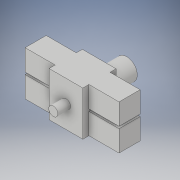
# Autodesk Inventor part: Semi Rotary Hydraulic Motor
Saved by Autodesk Inventor 2019 (Build 230136000, 136)
## iProperties
Created: 2020-09-30
Part Number: Semi Rotary Hydraulic Motor
Material: Generic
Document SubType Name: Modeling
Designer: Jawal
Density: 1 g/cm^3
Appearance: Default
Author: Jawal
Autodesk Inventor part; units mm, degrees
ref_plane "YZ Plane" through (0, 0, 0) normal (1, 0, 0) x (0, 1, 0)
ref_plane "XZ Plane" through (0, 0, 0) normal (0, 1, 0) x (-1, 0, 0)
ref_plane "XY Plane" through (0, 0, 0) normal (0, 0, 1) x (1, 0, 0)
sketch "Sketch1" plane through (0, 0, 0) normal (0, 0, 1) x (1, 0, 0)
  line L0 (-50.8, 66.75) -> (50.8, 66.75)
  line L1 (50.8, 66.75) -> (50.8, -66.6)
  line L2 (50.8, -66.6) -> (-50.8, -66.6)
  line L3 (-50.8, -66.6) -> (-50.8, 66.75)
  point P0 (0, 0)
  dimension "d1" = 101.6
  dimension "d2" = 133.35
  dimension "d3" = 66.75
  dimension "d4" = 50.8
  constraints: 8 end point, 2 parallel, 1 horizontal, 1 perpendicular
  measures "d1" distance of L0.start L0.end
  measures "d2" distance of L2.end L0.start
  measures "d3" distance from line of L0 point (0, 0)
  measures "d4" distance from line of L3 point (0, 0)
extrude "Extrusion1" add sketch "Sketch1" along normal blind 100.075
sketch "Sketch2" plane through (0, 0, 100.075) normal (0, 0, 1) x (1, 0, 0)
  circle A0 centre (0, 0) radius 13.625
  dimension "d7" = 27.25
  constraints: 1 centre point, 1 coincident
  measures "d7" diameter of A0
extrude "Extrusion2" add sketch "Sketch2" along normal blind 38.1
sketch "Sketch3" plane through (0, 0, 0) normal (0, 0, -1) x (-1, 0, 0)
  circle A0 centre (0, 0) radius 31.75
  dimension "d10" = 63.5
  constraints: 1 centre point, 1 coincident
  measures "d10" diameter of A0
extrude "Extrusion3" add sketch "Sketch3" along normal blind 82.55
sketch "Sketch4" plane through (50.8, -66.6, 0) normal (1, 0, 0) x (0, 0, -1)
  line L0 (0, 133.35) -> (-100.075, 133.35) projected
  line L1 (-81.787, 133.35) -> (-18.288, 133.35)
  line L2 (-18.288, 133.35) -> (-18.288, 69.851)
  line L3 (-18.288, 69.851) -> (-81.787, 69.851)
  line L4 (-81.787, 69.851) -> (-81.787, 133.35)
  line L5 (0, 133.35) -> (0, 0) projected
  line L6 (-100.075, 0) -> (-100.075, 133.35) projected
  line L7 (0, 0) -> (-100.075, 0) projected
  line L8 (-81.787, 0) -> (-18.288, 0)
  line L9 (-18.288, 0) -> (-18.288, 63.499)
  line L10 (-18.288, 63.499) -> (-81.787, 63.499)
  line L11 (-81.787, 63.499) -> (-81.787, 0)
  point P0 (0, 66.6)
  dimension "d13" = 18.288
  dimension "d14" = 18.288
  dimension "d15" = 63.499
  dimension "d16" = 63.499
  dimension "d17" = 63.499
  constraints: 16 end point, 4 parallel, 2 horizontal, 2 perpendicular, 2 point on line
  measures "d13" distance between parallel lines of L5 L2
  measures "d14" distance between parallel lines of L6 L4
  measures "d15" distance of L2.end L3.end
  measures "d16" distance of L3.end L1.start
  measures "d17" distance of L8.end L9.end
extrude "Extrusion4" add sketch "Sketch4" along normal blind 90.424 contours L2 L3 L4 L0 | L7 L11 L10 L9
sketch "Sketch5" plane through (-50.8, -66.6, 0) normal (-1, 0, 0) x (0, 0, 1)
  line L0 (18.288, 69.851) -> (18.288, 133.35) projected
  line L1 (18.288, 69.851) -> (81.787, 69.851) projected
  line L2 (18.288, 133.35) -> (81.787, 133.35)
  line L3 (81.787, 133.35) -> (81.787, 69.851)
  line L4 (81.787, 69.851) -> (18.288, 69.851)
  line L5 (18.288, 69.851) -> (18.288, 133.35)
  line L6 (18.288, 0) -> (18.288, 63.499) projected
  line L7 (81.787, 0) -> (81.787, 63.499) projected
  line L8 (18.288, 63.499) -> (81.787, 63.499)
  line L9 (81.787, 63.499) -> (81.787, 0)
  line L10 (81.787, 0) -> (18.288, 0)
  line L11 (18.288, 0) -> (18.288, 63.499)
  point P0 (0, 66.6)
  constraints: 16 end point, 4 parallel, 2 horizontal, 2 perpendicular
extrude "Extrusion5" add sketch "Sketch5" along normal blind 90.424
equation "\"d16\" = d15"
equation "\"d17\" = d15"
body "Solid1"
